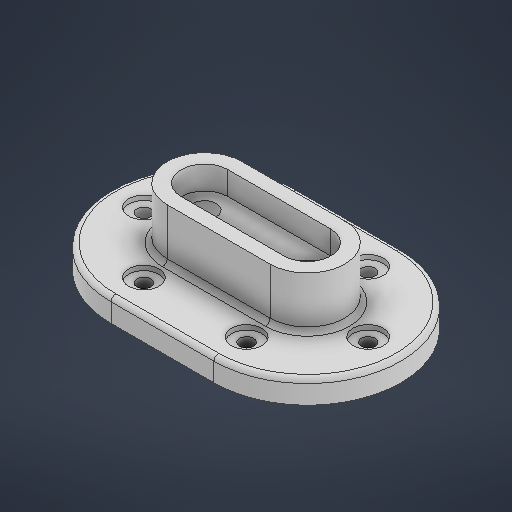
# Autodesk Inventor part: b2
Saved by Autodesk Inventor 2025.4 (Build 294407000, 407)
## iProperties
Created: 2026-05-18
Part Number: b2
Material: Generic
Document SubType Name: Modeling
Designer: VuQuan
Density: 1 g/cm^3
Appearance: Default
Author: VuQuan
Autodesk Inventor part; units mm, degrees
note: some values were not read from the file. Chosen so that the rebuilt part matches the saved one: direction of "Hole1"; direction of "Hole3".
ref_plane "YZ Plane" through (0, 0, 0) normal (1, 0, 0) x (0, 1, 0)
ref_plane "XZ Plane" through (0, 0, 0) normal (0, 1, 0) x (-1, 0, 0)
ref_plane "XY Plane" through (0, 0, 0) normal (0, 0, 1) x (1, 0, 0)
sketch "Sketch1" plane through (0, 0, 0) normal (0, 0, 1) x (1, 0, 0)
  line L0 (-22, 0) -> (22, 0) construction
  line L1 (-22, -40) -> (22, -40)
  line L2 (22, 40) -> (-22, 40)
  arc A0 (-22, 40) -> (-22, -40) centre (-22, 0) ccw
  arc A1 (22, -40) -> (22, 40) centre (22, 0) ccw
  line L3 (-22, 0) -> (22, 0) construction
  line L4 (-22, -16) -> (22, -16)
  line L5 (22, 16) -> (-22, 16)
  arc A2 (-22, 16) -> (-22, -16) centre (-22, 0) ccw
  arc A3 (22, -16) -> (22, 16) centre (22, 0) ccw
  line L6 (22, 10) -> (-22, 10)
  arc A4 (-22, 10) -> (-22, -10) centre (-22, 0) ccw
  line L7 (-22, -10) -> (22, -10)
  arc A5 (22, -10) -> (22, 10) centre (22, 0) ccw
  point P0 (0, 0)
  point P1 (0, 0)
  point P2 (62, 0)
  point P3 (-62, 0)
  point P4 (0, 0)
  point P5 (38, 0)
  point P6 (-38, 0)
  point P7 (-48, 0)
  point P8 (-22, -26)
  dimension "d1" = 124
  dimension "d2" = 76
  dimension "d3" = 80
  dimension "d4" = 16
  dimension "d5" = 10
  dimension "d6" = 26
  dimension "d7" = 26
  constraints: 20 end point, 16 point on circle, 8 tangent, 6 centre point, 4 equal length, 2 coincident, 2 midpoint, 1 horizontal, 1 point on line, 1 vertical alignment, 3 other
  measures "d1" distance of point (62, 0) point (-62, 0)
  measures "d2" distance of point (38, 0) point (-38, 0)
  measures "d3" distance between parallel lines of L2 L1
  measures "d4" radius of A3
  measures "d5" radius of A5
  measures "d6" distance of L3.start point (-48, 0)
  measures "d7" distance from line of L0 point (-22, -26)
extrude "Extrusion1" add sketch "Sketch1" along normal blind 10 contours A0 L2 A1 L1 | A2 L5 A3 L4 | A5 L7 A4 L6
extrude "Extrusion2" add sketch "Sketch1" along normal blind 32 contours A2 L5 A3 L4 | A5 L7 A4 L6
extrude "Extrusion3" cut sketch "Sketch1" against normal blind 10 from surface at 32 contours A5 L7 A4 L6
hole "Hole1" at (-22, -26, 0) at (-48, 0, 0) direction (0, 0, 1) diameter 6 depth 10
sketch "Sketch2" plane through (0, 0, 10) normal (0, 0, 1) x (1, 0, 0)
  circle A0 centre (-48, 0) radius 3 projected
  circle A1 centre (-22, -26) radius 3 projected
  point P0 (0, 0)
  constraints: 2 coincident
hole "Hole2" at (-48, 0, 10) at (-22, -26, 10) direction (0, 0, -1) diameter 13 depth 2
hole "Hole3" at (-22, 0, 0) direction (0, 0, 1) diameter 10 depth 22
mirror "Mirror1" about plane through (0, 0, 0) normal (1, 0, 0) of "Hole2", "Hole3", "Hole1"
mirror "Mirror2" about plane through (0, 0, 0) normal (0, 1, 0) of "Hole2", "Hole1", "Hole3", "Mirror1"
fillet "Fillet1" radius 2 8 edges at (62, 0, 10) (0, 40, 10) (-62, 0, 10) (0, -40, 10) (0, -16, 10) (-38, 0, 10) (0, 16, 10) (38, 0, 10)
move or copy body "Rotate1" bodies to move or copy 1 copy no rotation origin (0, 0, 0) rotation axis (1, 0, 0) rotation angle -90
body "Solid1"
